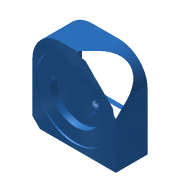
# Autodesk Inventor part: trim pot_ body
Saved by Autodesk Inventor 2014 (Build 180170000, 170)
## iProperties
Created: 2015-10-12
Part Number: trim pot_ body
Material: Generic
Document SubType Name: Modeling
Designer: Tom
Density: 1 g/cm^3
Appearance: Cyan
Author: Tom
Autodesk Inventor part; units mm, degrees
ref_plane "YZ Plane" through (0, 0, 0) normal (1, 0, 0) x (0, 1, 0)
ref_plane "XZ Plane" through (0, 0, 0) normal (0, 1, 0) x (-1, 0, 0)
ref_plane "XY Plane" through (0, 0, 0) normal (0, 0, 1) x (1, 0, 0)
sketch "Sketch1" plane through (0, 0, 0) normal (0, 0, 1) x (1, 0, 0)
  line L0 (-3.3401, -3.4417) -> (3.3401, -3.4417)
  line L1 (3.3401, -3.4417) -> (3.3401, 1.1557)
  line L2 (1.0541, 3.4417) -> (-1.0541, 3.4417)
  line L3 (-3.3401, 1.1557) -> (-3.3401, -3.4417)
  line L4 (-3.3401, -3.4417) -> (3.3401, 3.4417) construction
  line L5 (3.3401, -3.4417) -> (-3.3401, 3.4417) construction
  arc A0 (-1.0541, 3.4417) -> (-3.3401, 1.1557) centre (-1.0541, 1.1557) ccw
  arc A1 (3.3401, 1.1557) -> (1.0541, 3.4417) centre (1.0541, 1.1557) ccw
  point P0 (0, 0)
  dimension "d0" = 6.6802
  dimension "d1" = 6.8834
  dimension "d2" = 2.286
  constraints: 12 end point, 4 point on circle, 4 point on line, 4 tangent, 2 centre point, 2 midpoint, 2 parallel, 1 equal radius, 1 horizontal, 1 perpendicular
  measures "d0" distance of L5.end L4.end
  measures "d1" distance of L4.end L0.end
  measures "d2" radius of A0
extrude "Extrusion1" add sketch "Sketch1" along normal blind 2.54
sketch "Sketch2" plane through (0, 0, 2.54) normal (0, 0, 1) x (1, 0, 0)
  circle A0 centre (0, 0) radius 3.0734
  dimension "d5" = 6.1468
  constraints: 1 centre point, 1 coincident
  measures "d5" diameter of A0
extrude "Extrusion2" cut sketch "Sketch2" against normal blind 0.127
sketch "Sketch4" plane through (0, 0, 2.413) normal (0, 0, 1) x (1, 0, 0)
  circle A0 centre (0, 0) radius 3.0734 projected
  arc A1 (-1.9656, 0.4168) -> (1.9656, 0.4168) centre (0, 0) ccw
  arc A2 (-1.3084, 0.2505) -> (1.3084, 0.2505) centre (0, 0) ccw
  circle A3 centre (1.6419, 0.3144) radius 0.3175 projected
  line L0 (0, 0) -> (0, 0.9465)
  arc A4 (1.9656, 0.4168) -> (1.3084, 0.2505) centre (1.6419, 0.3144) ccw
  arc A5 (-1.3084, 0.2505) -> (-1.9656, 0.4168) centre (-1.6419, 0.3144) ccw
  dimension "d8" = 0.6772
  constraints: 8 point on circle, 4 centre point, 3 coincident, 3 symmetric about line, 2 end point, 1 tangent, 1 vertical, 1 other
  measures "d8" radial gap between concentric circles of A1 A2
extrude "Extrusion3" cut sketch "Sketch4" against normal blind 0.508 contours A5 A2 A4 A1
sketch "Sketch5" plane through (1.6419, 0.3144, 2.413) normal (0, 0, 1) x (1, 0, 0)
  circle A0 centre (0, 0) radius 0.3175 projected
  point P0 (-1.6419, -0.3144)
extrude "Extrusion4" cut sketch "Sketch5" against normal blind 0.508
sketch "Sketch6" plane through (0, 0, 0) normal (0, 0, -1) x (-1, 0, 0)
  line L0 (3.3401, 1.1557) -> (3.3401, -3.4417) projected
  line L1 (-1.0541, 3.4417) -> (1.0541, 3.4417) projected
  line L2 (-3.3401, -3.4417) -> (-3.3401, 1.1557) projected
  line L3 (-1.905, -1.0033) -> (1.905, -1.0033)
  line L4 (1.905, -1.0033) -> (1.905, 2.8067)
  line L5 (1.905, 2.8067) -> (-1.905, 2.8067)
  line L6 (-1.905, 2.8067) -> (-1.905, -1.0033)
  point P0 (0, 0)
  dimension "d13" = 3.81
  dimension "d14" = 3.81
  dimension "d15" = 6.6802
  dimension "d16" = 1.4351
  dimension "d17" = 0.635
  constraints: 8 end point, 2 parallel, 1 horizontal, 1 perpendicular
  measures "d13" distance of L5.end L4.end
  measures "d14" distance of L4.end L3.end
  measures "d15" distance between parallel lines of L2 L0
  measures "d16" horizontal distance of L2.end L5.end
  measures "d17" distance between parallel lines of L1 L5
extrude "Extrusion5" cut sketch "Sketch6" against normal blind 0.381
equation "\"d16\" = -0.5 * d13 + 0.5 * d15"
body "Solid1"
